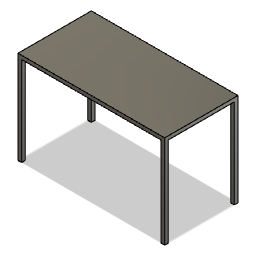
Table (Autodesk Fusion 360 design; units mm, degrees)
Autodesk Fusion 360 part; units mm, degrees
sketch "Sketch1" plane through (0, 0, 0) normal (0, 1, 0) x (1, 0, 0)
  line L0 (0, 0) -> (1200, 0)
  line L1 (1200, 0) -> (1200, 600)
  line L2 (1200, 600) -> (0, 600)
  line L3 (0, 600) -> (0, 0)
  constraint horizontal L0
  constraint vertical L1
  constraint horizontal L2
  constraint vertical L3
  constraint coincident L0.start L3.end
extrude "Extrude1" add sketch "Sketch1" along normal blind 30
sketch "Sketch2" plane through (0, 0, 0) normal (0, -1, 0) x (1, 0, 0)
  line L0 (0, 0) -> (0, -600)
  line L1 (0, -600) -> (1200, -600)
  line L2 (1200, -600) -> (1200, 0)
  line L3 (1200, 0) -> (0, 0)
  line L4 (0, 0) -> (30, 0)
  line L5 (30, 0) -> (30, -30)
  line L6 (30, -30) -> (0, -30)
  line L7 (0, -30) -> (0, 0)
  line L8 (0, -600) -> (30, -600)
  line L9 (30, -600) -> (30, -570)
  line L10 (30, -570) -> (0, -570)
  line L11 (0, -570) -> (0, -600)
  line L12 (1200, 0) -> (1170, 0)
  line L13 (1170, 0) -> (1170, -30)
  line L14 (1170, -30) -> (1200, -30)
  line L15 (1200, -30) -> (1200, 0)
  line L16 (1200, -600) -> (1170, -600)
  line L17 (1170, -600) -> (1170, -570)
  line L18 (1170, -570) -> (1200, -570)
  line L19 (1200, -570) -> (1200, -600)
  constraint horizontal L4
  constraint vertical L5
  constraint horizontal L6
  constraint vertical L7
  constraint coincident L0.start L3.end
  constraint horizontal L8
  constraint vertical L9
  constraint horizontal L10
  constraint vertical L11
  constraint coincident L0.end L1.start
  constraint horizontal L12
  constraint vertical L13
  constraint horizontal L14
  constraint vertical L15
  constraint coincident L2.end L3.start
  constraint horizontal L16
  constraint vertical L17
  constraint horizontal L18
  constraint vertical L19
  constraint coincident L1.end L2.start
extrude "Extrude2" add sketch "Sketch2" along normal blind 730 contours L0 L3 L4 L5 L6 L7 | L0 L1 L8 L9 L10 L11 | L2 L3 L12 L13 L14 L15 | L1 L2 L16 L17 L18 L19
